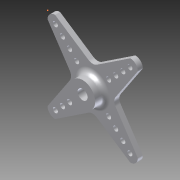
# Autodesk Inventor part: servoHornX
Saved by Autodesk Inventor 2012 (Build 160160000, 160)
## iProperties
Created: 2011-06-28
Part Number: servoHornX
Document SubType Name: Modeling
Designer: Byron
Density: 1 g/cm^3
Mass: 0.775055 g
Surface Area: 12.3226 cm^2
Volume: 0.775055 cm^3
Material: Default
Author: Byron
Autodesk Inventor part; units mm, degrees
ref_plane "YZ Plane" through (0, 0, 0) normal (1, 0, 0) x (0, 1, 0)
ref_plane "XZ Plane" through (0, 0, 0) normal (0, 1, 0) x (-1, 0, 0)
ref_plane "XY Plane" through (0, 0, 0) normal (0, 0, 1) x (1, 0, 0)
sketch "Sketch2" plane through (0, 0, 0) normal (0, 1, 0) x (-1, 0, 0)
  line L0 (-2.3812, 0) -> (-26.1937, 0) construction
  line L1 (-28.575, -2.3812) -> (-28.575, -26.1937) construction
  line L2 (-26.1937, -28.575) -> (-2.3812, -28.575) construction
  line L3 (0, -26.1937) -> (0, -2.3812) construction
  line L4 (-27.8023, -27.8024) -> (0.7727, 0.7726) construction
  line L5 (0, -28.575) -> (-28.575, 0) construction
  circle A0 centre (-14.2875, -14.2875) radius 6.35 construction
  line L6 (-14.2875, -28.575) -> (-14.2875, 0) construction
  line L7 (0, -14.2875) -> (-28.575, -14.2875) construction
  arc A1 (-2.3812, -28.575) -> (0, -26.1937) centre (-2.3812, -26.1937) ccw
  line L8 (0, -26.1937) -> (-7.0569, -15.6084)
  line L9 (-2.3812, -28.575) -> (-12.9666, -21.5181)
  arc A2 (-28.575, -26.1937) -> (-26.1937, -28.575) centre (-26.1937, -26.1937) ccw
  arc A3 (-26.1937, 0) -> (-28.575, -2.3812) centre (-26.1937, -2.3813) ccw
  arc A4 (0, -2.3812) -> (-2.3812, 0) centre (-2.3812, -2.3812) ccw
  line L10 (-15.6084, -21.5181) -> (-26.1937, -28.575)
  line L11 (-28.575, -26.1937) -> (-21.5181, -15.6084)
  line L12 (-21.5181, -12.9666) -> (-28.575, -2.3812)
  line L13 (-26.1937, 0) -> (-15.6084, -7.0569)
  line L14 (-12.9666, -7.0569) -> (-2.3812, 0)
  line L15 (0, -2.3812) -> (-7.0569, -12.9666)
  arc A5 (-12.9666, -21.5181) -> (-15.6084, -21.5181) centre (-14.2875, -23.4994) ccw
  arc A6 (-7.0569, -12.9666) -> (-7.0569, -15.6084) centre (-5.0756, -14.2875) ccw
  arc A7 (-15.6084, -7.0569) -> (-12.9666, -7.0569) centre (-14.2875, -5.0756) ccw
  arc A8 (-21.5181, -15.6084) -> (-21.5181, -12.9666) centre (-23.4994, -14.2875) ccw
  circle A9 centre (-26.0719, -26.072) radius 0.7938
  circle A10 centre (-14.2875, -14.2875) radius 16.6688 construction
  circle A11 centre (-23.8268, -23.8269) radius 0.7938
  circle A12 centre (-21.5818, -21.5819) radius 0.7938
  circle A13 centre (-19.3367, -19.3368) radius 0.7938
  circle A14 centre (-2.503, -26.0719) radius 0.7938
  circle A15 centre (-4.7481, -23.8268) radius 0.7938
  circle A16 centre (-6.9931, -21.5818) radius 0.7938
  circle A17 centre (-9.2382, -19.3367) radius 0.7938
  circle A18 centre (-2.5031, -2.503) radius 0.7938
  circle A19 centre (-4.7482, -4.7481) radius 0.7938
  circle A20 centre (-6.9932, -6.9931) radius 0.7938
  circle A21 centre (-9.2383, -9.2382) radius 0.7938
  circle A22 centre (-26.072, -2.5031) radius 0.7938
  circle A23 centre (-23.8269, -4.7482) radius 0.7938
  circle A24 centre (-21.5819, -6.9932) radius 0.7938
  circle A25 centre (-19.3368, -9.2383) radius 0.7938
  point P0 (0, 0)
  point P1 (-7.9375, -14.2875)
  point P2 (-14.2875, -20.6375)
  point P3 (-20.6375, -14.2875)
  point P4 (-14.2875, -7.9375)
  dimension "d0" = 27.813
  dimension "d1" = 27.8131
  dimension "d2" = 12.7
  dimension "d3" = 2.3813
  dimension "d4" = 2.3813
  dimension "d5" = 2.3813
  dimension "d6" = 1.5875
  dimension "d7" = 33.3375
  dimension "d10" = 3.175
  dimension "d17" = 360
  constraints: 32 end point, 26 centre point, 20 point on circle, 19 point on line, 16 tangent, 5 equal radius, 5 midpoint, 2 parallel, 1 coincident, 1 horizontal, 1 perpendicular, 40 other
  measures "d0" distance of L5.start L4.start
  measures "d1" distance of L5.end L4.start
  measures "d2" diameter of A0
  measures "d3" radius of A1
  measures "d4" radius of A2
  measures "d5" radius of A5
  measures "d6" diameter of A9
  measures "d7" diameter of A10
  measures "d10" distance of A9.centre A11.centre
extrude "Extrusion1" add sketch "Sketch2" along normal blind 1.5875
sketch "Sketch3" plane through (0, 0, 0) normal (0, -1, 0) x (1, 0, 0)
  circle A0 centre (14.2875, -14.2875) radius 3.9688
  circle A1 centre (14.2875, -14.2875) radius 1.5875
  point P0 (0, 0)
  dimension "d21" = 7.9375
  dimension "d22" = 3.175
  constraints: 2 centre point, 1 coincident
  measures "d21" diameter of A0
  measures "d22" diameter of A1
extrude "Extrusion2" add sketch "Sketch3" along normal blind 3.175
extrude "Extrusion3" cut sketch "Sketch3" against normal through all contours A1
fillet "Fillet1" radius 1.5875 1 edges at (10.3187, 0, -14.2875)
body "Solid1"
